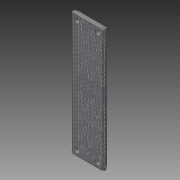
# Autodesk Inventor part: ESP_DISP_BACK
Saved by Autodesk Inventor 2015 (Build 190159000, 159)
## iProperties
Created: 2018-04-03
Part Number: ESP_DISP_BACK
Material: Типовые
Document SubType Name: Modeling
Designer: JOK
Density: 1 g/cm^3
Appearance: По умолчанию
Author: JOK
Autodesk Inventor part; units mm, degrees
ref_plane "YZ Plane" through (0, 0, 0) normal (1, 0, 0) x (0, 1, 0)
ref_plane "XZ Plane" through (0, 0, 0) normal (0, 1, 0) x (-1, 0, 0)
ref_plane "XY Plane" through (0, 0, 0) normal (0, 0, 1) x (1, 0, 0)
sketch "Эскиз1" plane through (0, 0, 0) normal (0, 1, 0) x (-1, 0, 0)
  line L0 (-20, 90) -> (20, 90)
  line L1 (20, 90) -> (20, -90)
  line L2 (20, -90) -> (-20, -90)
  line L3 (-20, -90) -> (-20, 90)
  line L4 (-20, 90) -> (20, -90) construction
  line L5 (20, 90) -> (-20, -90) construction
  line L6 (16, -86) -> (-16, -86)
  line L7 (-16, -86) -> (-16, 86)
  line L8 (-16, 86) -> (16, 86)
  line L9 (16, 86) -> (16, -86)
  line L10 (16, -86) -> (-16, 86) construction
  line L11 (-16, -86) -> (16, 86) construction
  line L12 (-11, 74) -> (11, 74)
  line L13 (11, 74) -> (11, -74)
  line L14 (11, -74) -> (-11, -74)
  line L15 (-11, -74) -> (-11, 74)
  line L16 (-11, 74) -> (11, -74) construction
  line L17 (11, 74) -> (-11, -74) construction
  circle A0 centre (16, 86) radius 1.6
  line L18 (17.7, 80.7) -> (-17.7, 80.7)
  line L19 (-17.7, 80.7) -> (-17.7, -80.7)
  line L20 (-17.7, -80.7) -> (17.7, -80.7)
  line L21 (17.7, -80.7) -> (17.7, 80.7)
  line L22 (17.7, 80.7) -> (-17.7, -80.7) construction
  line L23 (-17.7, 80.7) -> (17.7, -80.7) construction
  line L24 (-8.89, -88.5) -> (8.89, -88.5)
  line L25 (8.89, -88.5) -> (8.89, -83.5)
  line L26 (8.89, -83.5) -> (-8.89, -83.5)
  line L27 (-8.89, -83.5) -> (-8.89, -88.5)
  line L28 (-8.89, -88.5) -> (8.89, -83.5) construction
  line L29 (8.89, -88.5) -> (-8.89, -83.5) construction
  point P0 (0, 0)
  point P1 (0, -86)
  dimension "d0" = 40
  dimension "d1" = 180
  dimension "d2" = 32
  dimension "d3" = 172
  dimension "d4" = 22
  dimension "d5" = 148
  dimension "d6" = 3.2
  dimension "d7" = 35.4
  dimension "d8" = 161.4
  dimension "d21" = 17.78
  dimension "d22" = 5
  constraints: 60 end point, 11 midpoint, 10 parallel, 5 coincident, 5 horizontal, 5 perpendicular, 1 centre point
  measures "d0" distance of L1.end L2.end
  measures "d1" distance of L0.end L1.end
  measures "d2" distance of L7.end L8.end
  measures "d3" distance of L6.end L7.end
  measures "d4" distance of L13.end L14.end
  measures "d5" distance of L12.end L13.end
  measures "d6" diameter of A0
  measures "d7" distance of L20.end L19.end
  measures "d8" distance of L19.end L18.end
  measures "d21" distance of L26.end L25.end
  measures "d22" distance of L25.end L24.end
sketch "Эскиз17" plane through (0, 0, 0) normal (0, 1, 0) x (-1, 0, 0)
  line L0 (-25, 95) -> (25, 95)
  line L1 (25, 95) -> (25, -95)
  line L2 (25, -95) -> (-25, -95)
  line L3 (-25, -95) -> (-25, 95)
  line L4 (-25, 95) -> (25, -95) construction
  line L5 (25, 95) -> (-25, -95) construction
  point P0 (0, 0)
  dimension "d92" = 50
  dimension "d93" = 190
  constraints: 12 end point, 2 midpoint, 2 parallel, 1 horizontal, 1 perpendicular
  measures "d92" distance of L1.end L2.end
  measures "d93" distance of L0.end L1.end
extrude "Выдавливание17" add sketch "Эскиз17" along normal blind 4
sketch "Эскиз18" plane through (0, 4, 0) normal (0, 1, 0) x (1, 0, 0)
  line L0 (22, -92) -> (-22, -92)
  line L1 (-22, -92) -> (-22, 92)
  line L2 (-22, 92) -> (22, 92)
  line L3 (22, 92) -> (22, -92)
  line L4 (22, -92) -> (-22, 92) construction
  line L5 (-22, -92) -> (22, 92) construction
  point P0 (0, 0)
  dimension "d96" = 44
  dimension "d97" = 184
  constraints: 12 end point, 2 midpoint, 2 parallel, 1 horizontal, 1 perpendicular
  measures "d96" distance of L1.end L2.end
  measures "d97" distance of L0.end L1.end
extrude "Выдавливание18" add sketch "Эскиз18" along normal blind 4
sketch "Эскиз19" plane through (0, 8, 0) normal (0, 1, 0) x (1, 0, 0)
  line L0 (17.5, -87.5) -> (-17.5, -87.5)
  line L1 (-17.5, -87.5) -> (-17.5, 87.5)
  line L2 (-17.5, 87.5) -> (17.5, 87.5)
  line L3 (17.5, 87.5) -> (17.5, -87.5)
  line L4 (17.5, -87.5) -> (-17.5, 87.5) construction
  line L5 (-17.5, -87.5) -> (17.5, 87.5) construction
  point P0 (0, 0)
  dimension "d100" = 35
  dimension "d101" = 175
  constraints: 12 end point, 2 midpoint, 2 parallel, 1 horizontal, 1 perpendicular
  measures "d100" distance of L1.end L2.end
  measures "d101" distance of L0.end L1.end
extrude "Выдавливание19" cut sketch "Эскиз19" against normal blind 4
sketch "Эскиз20" plane through (0, 0, 0) normal (0, -1, 0) x (1, 0, 0)
  point P0 (0, 0)
  point P1 (16, 86)
  point P2 (-16, 86)
  point P3 (-16, -86)
  point P4 (16, -86)
sketch "Эскиз21" plane through (0, 4, 0) normal (0, 1, 0) x (1, 0, 0)
  circle A0 centre (-16, -86) radius 4
  circle A1 centre (16, -86) radius 4
  circle A2 centre (16, 86) radius 4
  circle A3 centre (-16, 86) radius 4
  point P0 (0, 0)
  dimension "d104" = 8
  dimension "d105" = 8
  constraints: 4 centre point
  measures "d104" diameter of A2
  measures "d105" diameter of A3
sketch "Эскиз22" plane through (0, 4, 0) normal (0, 1, 0) x (1, 0, 0)
  line L0 (-17.5, -87.5) -> (-17.5, 87.5) projected
  line L1 (17.5, 2) -> (-17.5, 2)
  line L2 (-17.5, 2) -> (-17.5, -2)
  line L3 (-17.5, -2) -> (17.5, -2)
  line L4 (17.5, -2) -> (17.5, 2)
  line L5 (17.5, 2) -> (-17.5, -2) construction
  line L6 (-17.5, 2) -> (17.5, -2) construction
  line L7 (-17.5, 87.5) -> (17.5, 87.5) projected
  line L8 (-2, -87.5) -> (2, -87.5)
  line L9 (2, -87.5) -> (2, 87.5)
  line L10 (2, 87.5) -> (-2, 87.5)
  line L11 (-2, 87.5) -> (-2, -87.5)
  line L12 (-2, -87.5) -> (2, 87.5) construction
  line L13 (2, -87.5) -> (-2, 87.5) construction
  line L14 (-17.5, 2) -> (-2, 87.5) construction
  line L15 (-15.5321, 1.6432) -> (-0.0321, 87.1432)
  line L16 (-3.9679, 87.8568) -> (-19.4679, 2.3568)
  arc A0 (-19.4679, 2.3568) -> (-15.5321, 1.6432) centre (-17.5, 2) ccw
  arc A1 (-0.0321, 87.1432) -> (-3.9679, 87.8568) centre (-2, 87.5) ccw
  line L17 (-17.5, 87.5) -> (-2, 2) construction
  line L18 (-19.4679, 87.1432) -> (-3.9679, 1.6432)
  line L19 (-0.0321, 2.3568) -> (-15.5321, 87.8568)
  arc A2 (-15.5321, 87.8568) -> (-19.4679, 87.1432) centre (-17.5, 87.5) ccw
  arc A3 (-3.9679, 1.6432) -> (-0.0321, 2.3568) centre (-2, 2) ccw
  line L20 (2, 2) -> (17.5, 87.5) construction
  line L21 (3.9679, 1.6432) -> (19.4679, 87.1432)
  line L22 (15.5321, 87.8568) -> (0.0321, 2.3568)
  arc A4 (0.0321, 2.3568) -> (3.9679, 1.6432) centre (2, 2) ccw
  arc A5 (19.4679, 87.1432) -> (15.5321, 87.8568) centre (17.5, 87.5) ccw
  line L23 (17.5, 2) -> (2, 87.5) construction
  line L24 (19.4679, 2.3568) -> (3.9679, 87.8568)
  line L25 (0.0321, 87.1432) -> (15.5321, 1.6432)
  arc A6 (15.5321, 1.6432) -> (19.4679, 2.3568) centre (17.5, 2) ccw
  arc A7 (3.9679, 87.8568) -> (0.0321, 87.1432) centre (2, 87.5) ccw
  line L26 (17.5, -87.5) -> (2, -2) construction
  line L27 (19.4679, -87.1432) -> (3.9679, -1.6432)
  line L28 (0.0321, -2.3568) -> (15.5321, -87.8568)
  arc A8 (15.5321, -87.8568) -> (19.4679, -87.1432) centre (17.5, -87.5) ccw
  arc A9 (3.9679, -1.6432) -> (0.0321, -2.3568) centre (2, -2) ccw
  line L29 (-17.5, -87.5) -> (-2, -2) construction
  line L30 (-15.5321, -87.8568) -> (-0.0321, -2.3568)
  line L31 (-3.9679, -1.6432) -> (-19.4679, -87.1432)
  arc A10 (-19.4679, -87.1432) -> (-15.5321, -87.8568) centre (-17.5, -87.5) ccw
  arc A11 (-0.0321, -2.3568) -> (-3.9679, -1.6432) centre (-2, -2) ccw
  line L32 (-17.5, -2) -> (-2, -87.5) construction
  line L33 (-19.4679, -2.3568) -> (-3.9679, -87.8568)
  line L34 (-0.0321, -87.1432) -> (-15.5321, -1.6432)
  arc A12 (-15.5321, -1.6432) -> (-19.4679, -2.3568) centre (-17.5, -2) ccw
  arc A13 (-3.9679, -87.8568) -> (-0.0321, -87.1432) centre (-2, -87.5) ccw
  line L35 (17.5, -2) -> (2, -87.5) construction
  line L36 (15.5321, -1.6432) -> (0.0321, -87.1432)
  line L37 (3.9679, -87.8568) -> (19.4679, -2.3568)
  arc A14 (19.4679, -2.3568) -> (15.5321, -1.6432) centre (17.5, -2) ccw
  arc A15 (0.0321, -87.1432) -> (3.9679, -87.8568) centre (2, -87.5) ccw
  point P0 (0, 0)
  point P1 (-9.75, 44.75)
  point P2 (-9.75, 44.75)
  point P3 (9.75, 44.75)
  point P4 (9.75, 44.75)
  point P5 (9.75, -44.75)
  point P6 (-9.75, -44.75)
  point P7 (-9.75, -44.75)
  point P8 (9.75, -44.75)
  dimension "d106" = 4
  dimension "d107" = 4
  dimension "d108" = 4
  dimension "d109" = 4
  dimension "d110" = 4
  dimension "d111" = 4
  dimension "d112" = 4
  dimension "d113" = 4
  constraints: 89 end point, 32 point on circle, 32 tangent, 16 centre point, 15 parallel, 12 midpoint, 10 point on line, 2 horizontal, 2 perpendicular
  measures "d106" diameter of A1
  measures "d107" diameter of A3
  measures "d108" diameter of A5
  measures "d109" diameter of A7
  measures "d110" diameter of A9
  measures "d111" diameter of A11
  measures "d112" diameter of A13
  measures "d113" diameter of A15
extrude "Выдавливание20" add sketch "Эскиз22" along normal blind 4 contours L31 L33 L30 A10 | L33 A12 L0 | L0 L3 L34 L31 L33 | L31 L34 L30 L33 | L0 A12 L34 L3 | L31 L3 L11 L30 L34 | L30 L34 L11 L8 A13 L33 | A0 L16 L0 | L0 L1 L15 A0 | A0 L15 L1 L18 A3 A11 L31 L3 L34 A12 | L31 A11 L11 L3 | L0 L16 L18 L15 L1 | L11 A11 L3 | L3 A11 L30 L11 | L30 A11 A9 L28 L9 L36 A15 A13 L34 L11 | L34 A13 L8 L11 | A15 L36 L9 L8 | L8 L9 L36 L28 L37 A15 | A9 L9 L3 | A11 A3 A4 A9 | L3 L9 L28 A9 | A3 L18 L1 L11 | L11 L1 A3 | L18 A2 L19 L7 L0 | L0 L7 L19 L16 L18 | L16 L19 L15 L18 | L18 L15 L19 L11 L1 | L9 A9 L27 L3 | L3 L27 L36 L28 L9 | A4 L1 L9 | L9 L1 L21 A4 | A4 L21 L1 L25 A6 A14 L36 L3 L27 A9 | L11 L19 A3 L1 | A4 L22 L9 L1 | A3 L19 L11 L15 A1 A7 L25 L9 L22 A4 | L37 L27 A8 L28 | L28 L36 L27 L37 | L16 L7 L11 L15 L19 | L9 L22 L25 L21 L1 | L27 L36 L3 L4 A14 L37 | L16 A1 L7 | L11 L7 A1 L15 | L36 A14 L4 L3 | L25 L21 L24 A6 L4 L1 | L1 L4 A6 L25 | L25 L22 L24 L21 | L25 A7 L7 L9 | L9 L7 L24 L22 L25 | A7 L24 L7 | L24 L22 A5 L21
extrude "Выдавливание21" add sketch "Эскиз21" along normal blind 4
hole "Отверстие1" at (16, 0, 86) at (-16, 0, 86) at (-16, 0, -86) at (16, 0, -86) direction (0, 1, 0) diameter 3.2 end through all countersink diameter 8 countersink angle 90
sketch "Эскиз23" plane through (0, 4, 0) normal (0, 1, 0) x (1, 0, 0)
  line L0 (17.5, 42.75) -> (-17.5, 42.75)
  line L1 (-17.5, 42.75) -> (-17.5, 46.75)
  line L2 (-17.5, 46.75) -> (17.5, 46.75)
  line L3 (17.5, 46.75) -> (17.5, 42.75)
  line L4 (17.5, 42.75) -> (-17.5, 46.75) construction
  line L5 (-17.5, 42.75) -> (17.5, 46.75) construction
  line L6 (-17.5, -42.75) -> (17.5, -42.75)
  line L7 (17.5, -42.75) -> (17.5, -46.75)
  line L8 (17.5, -46.75) -> (-17.5, -46.75)
  line L9 (-17.5, -46.75) -> (-17.5, -42.75)
  line L10 (-17.5, -42.75) -> (17.5, -46.75) construction
  line L11 (17.5, -42.75) -> (-17.5, -46.75) construction
  point P0 (0, 0)
  point P1 (0, 44.75)
  point P2 (0, -44.75)
  dimension "d125" = 35
  dimension "d126" = 4
  dimension "d127" = 35
  dimension "d128" = 4
  constraints: 24 end point, 4 midpoint, 4 parallel, 2 horizontal, 2 perpendicular
  measures "d125" distance of L1.end L2.end
  measures "d126" distance of L0.end L1.end
  measures "d127" distance of L7.end L8.end
  measures "d128" distance of L6.end L7.end
extrude "Выдавливание22" add sketch "Эскиз23" along normal blind 4
fillet "Сопряжение6" radius 3 4 edges at (-25, 2, 95) (25, 2, 95) (25, 2, -95) (-25, 2, -95)
fillet "Сопряжение7" radius 2 8 edges at (24.1213, 0, 94.1213) (0, 0, 95) (-24.1213, 0, 94.1213) (-25, 0, 0) (-24.1213, 0, -94.1213) (0, 0, -95) (24.1213, 0, -94.1213) (25, 0, 0)
